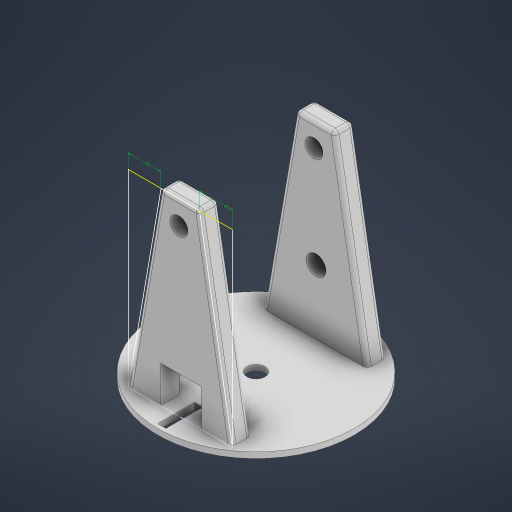
# Autodesk Inventor part: turret-base
Saved by Autodesk Inventor 2023 (Build 270158000, 158)
## iProperties
Created: 2022-05-15
Part Number: turret-base
Material: Generic
Document SubType Name: Modeling
Designer: jayso
Density: 1 g/cm^3
Appearance: Default
Author: jayso
Autodesk Inventor part; units mm, degrees
ref_plane "YZ Plane" through (0, 0, 0) normal (1, 0, 0) x (0, 1, 0)
ref_plane "XZ Plane" through (0, 0, 0) normal (0, 1, 0) x (-1, 0, 0)
ref_plane "XY Plane" through (0, 0, 0) normal (0, 0, 1) x (1, 0, 0)
sketch "Sketch1" plane through (0, 0, 0) normal (0, 1, 0) x (-1, 0, 0)
  circle A0 centre (0, 0) radius 120
  dimension "d0" = 240
  constraints: 1 centre point, 1 coincident
  measures "d0" diameter of A0
extrude "Extrusion1" add sketch "Sketch1" along normal blind 7
sketch "Sketch2" plane through (0, 7, 0) normal (0, 1, 0) x (1, 0, 0)
  circle A0 centre (0, 0) radius 11
  dimension "d3" = 22
  constraints: 1 centre point, 1 coincident
  measures "d3" diameter of A0
extrude "Extrusion2" cut sketch "Sketch2" against normal blind 7
sketch "Sketch4" plane through (0, 7, 0) normal (0, 1, 0) x (1, 0, 0)
  circle A0 centre (0, 0) radius 120 projected
  line L0 (-4.9843, -70) -> (5.0157, -70)
  line L1 (5.0157, -70) -> (5.0157, -115)
  line L2 (5.0157, -115) -> (-4.9843, -115)
  line L3 (-4.9843, -115) -> (-4.9843, -70)
  circle A1 centre (0, 0) radius 11 projected
  circle A2 centre (0, 0) radius 120 projected
  point P0 (0.0157, -70)
  point P1 (0, -120)
  dimension "d51" = 45
  dimension "d52" = 10
  dimension "d53" = 70
  constraints: 8 end point, 2 parallel, 1 horizontal, 1 midpoint, 1 perpendicular, 1 vertical alignment, 1 other
  measures "d51" distance of L0.end L1.end
  measures "d52" distance of L0.start L0.end
  measures "d53" distance of A1.centre point (0.016, -70)
sketch "Sketch5" plane through (0, 7, 0) normal (0, 1, 0) x (1, 0, 0)
  line L0 (-62.1079, -94) -> (64.8921, -94)
  line L1 (64.8921, -94) -> (64.8921, -71)
  line L2 (64.8921, -71) -> (-62.1079, -71)
  line L3 (-62.1079, -71) -> (-62.1079, -94)
  circle A0 centre (0, -94) radius 5 projected
  point P0 (0, 0)
  point P1 (-5, -94)
  point P2 (5, -94)
  dimension "d10" = 127
  dimension "d11" = 23
  dimension "d12" = 5
  constraints: 8 end point, 2 parallel, 1 horizontal, 1 perpendicular
  measures "d10" distance of L2.end L1.end
  measures "d11" distance of L0.end L1.end
  measures "d12" distance edge to line of A0 L0
sketch "Sketch6" plane through (0, 7, 0) normal (0, 1, 0) x (1, 0, 0)
  line L0 (-62.1079, 71) -> (64.8921, 71)
  line L1 (64.8921, 71) -> (64.8921, 94)
  line L2 (64.8921, 94) -> (-62.1079, 94)
  line L3 (-62.1079, 94) -> (-62.1079, 71)
  circle A0 centre (0, 0) radius 11 projected
  point P0 (1.3921, 71)
  dimension "d13" = 127
  dimension "d14" = 23
  dimension "d16" = 71
  constraints: 8 end point, 2 parallel, 1 horizontal, 1 midpoint, 1 perpendicular
  measures "d13" distance of L2.end L1.end
  measures "d14" distance of L0.end L1.end
  measures "d16" vertical distance of point (1.392, 71) A0.centre
extrude "Extrusion4" add sketch "Sketch5" along normal blind 230 contours A0 L0 L3 L2 L1
extrude "Extrusion5" add sketch "Sketch6" along normal blind 230 contours L3 L2 L1 L0
sketch "Sketch7" plane through (64.8921, 7, 71) normal (0, 0, -1) x (-1, 0, 0)
  line L0 (127, 0) -> (0, 0) projected
  line L1 (87.3921, 0) -> (37.3921, 0)
  line L2 (37.3921, 0) -> (37.3921, 45)
  line L3 (37.3921, 45) -> (87.3921, 45)
  line L4 (87.3921, 45) -> (87.3921, 0)
  line L5 (53.8921, 0) -> (75.8921, 0) projected
  line L6 (64.8921, 0) -> (64.8921, 26.8909)
  point P0 (64.8921, -7)
  point P1 (87.3921, 22.5)
  dimension "d21" = 50
  dimension "d22" = 45
  dimension "d23" = 22.5
  constraints: 10 end point, 2 midpoint, 2 parallel, 1 horizontal, 1 perpendicular, 1 point on line, 1 vertical
  measures "d21" distance of L2.end L3.end
  measures "d22" distance of L2.end L1.end
  measures "d23" distance from line of L6 point (87.392, 22.5)
extrude "Extrusion6" cut sketch "Sketch7" against normal blind 230
sketch "Sketch8" plane through (0, 237, 0) normal (0, 1, 0) x (1, 0, 0)
  arc A0 (5, -94) -> (-5, -94) centre (0, -94) ccw projected
  line L0 (5, -94) -> (64.8921, -94) projected
  arc A1 (0, -89) -> (5, -94) centre (0, -94) ccw
  line L1 (-62.1079, -94) -> (-5, -94) projected
  line L2 (5, -94) -> (-5, -94)
  point P0 (0, 0)
  constraints: 4 point on circle, 2 end point, 1 centre point, 1 horizontal
extrude "Extrusion7" add sketch "Sketch8" against normal blind 185 contours L2 A0
sketch "Sketch9" plane through (-62.1079, 237, 94) normal (0, 0, 1) x (1, 0, 0)
  line L0 (127, -230) -> (89.6079, -230) projected
  line L1 (127, -230) -> (87, 0)
  line L2 (127, 0) -> (0, 0) projected
  line L3 (39.6079, -230) -> (0, -230) projected
  line L4 (0, -230) -> (40, 0)
  line L5 (40, 0) -> (87, 0)
  line L6 (40, 0) -> (87, 0)
  point P0 (62.1079, -237)
  dimension "d28" = 40
  dimension "d29" = 40
  constraints: 8 end point, 1 collinear, 1 horizontal, 1 point on line
  measures "d28" distance of L2.end L4.end
  measures "d29" distance of L2.start L1.end
sketch "Sketch10" plane through (-62.1079, 237, 94) normal (0, 0, 1) x (1, 0, 0)
  line L0 (0, -230) -> (0, 0) projected
  line L1 (0, 0) -> (0, -230)
  line L2 (127, -230) -> (127, 0) projected
  line L3 (0, -230) -> (127, -230)
  line L4 (127, -230) -> (127, 0)
  point P0 (62.1079, -237)
  constraints: 6 end point, 2 collinear, 1 perpendicular
sketch "Sketch11" plane through (64.8921, 7, -94) normal (0, 0, -1) x (-1, 0, 0)
  line L0 (0, 0) -> (40, 230)
  line L1 (0, 230) -> (127, 230) projected
  line L2 (87.3921, 0) -> (127, 0) projected
  line L3 (127, 0) -> (87, 230)
  line L4 (87, 230) -> (40, 230)
  line L5 (127, 0) -> (127, 230) projected
  line L6 (0, 0) -> (0, 230) projected
  line L7 (0, 0) -> (0, 230)
  line L8 (0, 230) -> (40, 230)
  line L9 (127, 0) -> (127, 230)
  line L10 (127, 230) -> (87, 230)
  point P0 (64.8921, -7)
  dimension "d30" = 40
  dimension "d31" = 40
  constraints: 14 end point, 3 perpendicular, 2 point on line, 1 collinear
  measures "d30" distance of L0.end L1.start
  measures "d31" distance of L1.end L3.end
extrude "Extrusion8" cut sketch "Sketch11" against normal blind 277.075
fillet "Fillet1" radius 5 8 edges at (44.8921, 122, -94) (1.3921, 237, -94) (-42.1079, 122, -94) (-42.1079, 122, -71) (1.3921, 237, -71) (44.8921, 122, -71) (24.8921, 237, -82.5) (-22.1079, 237, -82.5)
fillet "Fillet2" radius 5 8 edges at (-42.1079, 122, 94) (-42.1079, 122, 71) (1.3921, 237, 94) (44.8921, 122, 94) (44.8921, 122, 71) (24.8921, 237, 82.5) (-22.1079, 237, 82.5) (1.3921, 237, 71)
sketch "Sketch12" plane through (-22.5, 52, 94) normal (0, 0, 1) x (1, 0, 0)
  circle A0 centre (22.5, 156.0331) radius 11
  point P0 (22.5, -52)
  dimension "d36" = 22
  constraints: 1 centre point
  measures "d36" diameter of A0
extrude "Extrusion9" cut sketch "Sketch12" against normal blind 277.075
sketch "Sketch13" plane through (59.8171, 7, -94) normal (0, 0, -1) x (-1, 0, 0)
  line L0 (32.3171, 56.0331) -> (32.3171, 101.0331)
  line L1 (82.3171, 101.0331) -> (82.3171, 56.0331)
  line L2 (32.3171, 101.0331) -> (82.3171, 101.0331)
  line L3 (82.3171, 101.0331) -> (82.3171, 56.0331)
  line L4 (82.3171, 56.0331) -> (32.3171, 56.0331)
  line L5 (32.3171, 56.0331) -> (32.3171, 101.0331)
  circle A0 centre (59.8171, 201.0331) radius 11 projected
  point P0 (59.8171, -7)
  point P1 (82.3171, 101.0331)
  point P2 (57.3171, 101.0331)
  dimension "d45" = 100
  constraints: 12 end point, 1 midpoint
  measures "d45" vertical distance of A0.centre point (57.317, 101.033)
extrude "Extrusion10" cut sketch "Sketch13" against normal blind 7 contours L0 L2 L1 L4
sketch "Sketch16" plane through (-57.0328, 7, -71) normal (0, 0, 1) x (1, 0, 0)
  point P0 (57.0328, -7)
sketch "Sketch17" plane through (59.8171, 7, -87) normal (0, 0, -1) x (-1, 0, 0)
  circle A0 centre (57.3171, 78.5331) radius 12
  line L0 (32.3171, 101.0331) -> (82.3171, 101.0331) projected
  line L1 (82.3171, 101.0331) -> (82.3171, 56.0331) projected
  point P0 (59.8171, -7)
  point P1 (57.3171, 101.0331)
  dimension "d46" = 24
  dimension "d47" = 22.5
  dimension "d48" = 25
  constraints: 1 centre point, 1 midpoint
  measures "d46" diameter of A0
  measures "d47" distance of point (57.317, 101.033) A0.centre
  measures "d48" distance from line of L1 A0.centre
extrude "Extrusion12" cut sketch "Sketch17" against normal blind 16
extrude "Extrusion13" cut sketch "Sketch4" against normal blind 10 contours L0 L1 L2 L3
body "Solid1"
